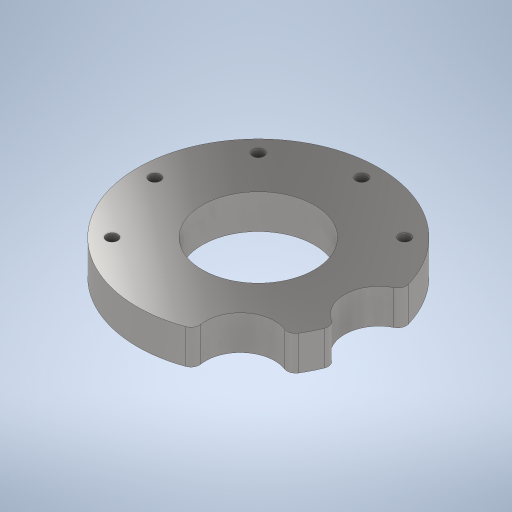
# Autodesk Inventor part: Weapon Hub Support
Saved by Autodesk Inventor 2023 (Build 270158000, 158)
## iProperties
Created: 2021-11-28
Part Number: Weapon Hub Support
Material: Steel, Carbon
Document SubType Name: Modeling
Designer: karen
Density: 7.85 g/cm^3
Appearance: Semi-Polished
Author: karen
Autodesk Inventor part; units mm, degrees
ref_plane "YZ Plane" through (0, 0, 0) normal (1, 0, 0) x (0, 1, 0)
ref_plane "XZ Plane" through (0, 0, 0) normal (0, 1, 0) x (-1, 0, 0)
ref_plane "XY Plane" through (0, 0, 0) normal (0, 0, 1) x (1, 0, 0)
sketch "Sketch1" plane through (0, 0, 0) normal (0, 1, 0) x (-1, 0, 0)
  circle A0 centre (0, 0) radius 44.45
  dimension "d0" = 88.9
  constraints: 1 centre point, 1 coincident
  measures "d0" diameter of A0
extrude "Extrusion1" add sketch "Sketch1" along normal blind 12.7
sketch "Sketch2" plane through (0, 12.7, 0) normal (0, 1, 0) x (1, 0, 0)
  circle A0 centre (0, 0) radius 19.05
  dimension "d3" = 38.1
  constraints: 1 centre point, 1 coincident
  measures "d3" diameter of A0
extrude "Extrusion2" cut sketch "Sketch2" against normal blind 12.7
sketch "Sketch4" plane through (0, 12.7, 0) normal (0, 1, 0) x (1, 0, 0)
  circle A0 centre (0, 0) radius 20.6375
  dimension "d17" = 41.275
  constraints: 1 centre point, 1 coincident
  measures "d17" diameter of A0
extrude "Extrusion4" cut sketch "Sketch4" against normal blind 25.4
sketch "Sketch5" plane through (0, 12.7, 0) normal (0, 1, 0) x (1, 0, 0)
  line L0 (0, 0) -> (0, 38.1)
  line L1 (0, 0) -> (26.9408, 26.9408)
  line L2 (0, 0) -> (-26.9408, 26.9408)
  line L3 (0, 0) -> (-38.1, 0)
  line L4 (0, 0) -> (-26.9408, -26.9408)
  circle A0 centre (0, 38.1) radius 2.0828
  circle A1 centre (26.9408, 26.9408) radius 2.0828
  circle A2 centre (-26.9408, 26.9408) radius 2.0828
  circle A3 centre (-38.1, 0) radius 2.0828
  circle A4 centre (-26.9408, -26.9408) radius 2.0828
  dimension "d20" = 38.1
  dimension "d21" = 38.1
  dimension "d22" = 45
  dimension "d23" = 38.1
  dimension "d24" = 45
  dimension "d25" = 38.1
  dimension "d26" = 38.1
  dimension "d27" = 45
  dimension "d28" = 4.1656
  dimension "d29" = 4.1656
  dimension "d30" = 4.1656
  dimension "d31" = 4.1656
  dimension "d32" = 4.1656
  constraints: 10 end point, 5 centre point, 4 coincident, 1 horizontal, 1 point on line, 1 vertical
  measures "d20" distance of L0.start L0.end
  measures "d21" distance of L0.start L1.end
  measures "d22" angle of L0 L1
  measures "d23" distance of L0.start L2.end
  measures "d24" angle of L0 L2
  measures "d25" distance of L0.start L3.end
  measures "d26" distance of L0.start L4.end
  measures "d27" angle of L3 L4
  measures "d28" diameter of A0
  measures "d29" diameter of A1
  measures "d30" diameter of A2
  measures "d31" diameter of A3
  measures "d32" diameter of A4
extrude "Extrusion5" cut sketch "Sketch5" against normal blind 12.7
sketch "Sketch6" plane through (0, 12.7, 0) normal (0, 1, 0) x (1, 0, 0)
  circle A0 centre (46.8049, -2.3327) radius 4.7625
  circle A1 centre (26.9408, 26.9408) radius 2.0828 projected
  point P0 (0, 0)
  dimension "d35" = 9.525
  dimension "d36" = 46.863
  dimension "d39" = 29.2735
  constraints: 1 centre point
  measures "d35" diameter of A0
  measures "d36" distance of point (0, 0) A0.centre
  measures "d39" vertical distance of A1.centre A0.centre
extrude "Extrusion6" cut sketch "Sketch6" against normal blind 12.7 contours A0
sketch "Sketch7" plane through (0, 12.7, 0) normal (0, 1, 0) x (1, 0, 0)
  circle A0 centre (29.6672, -36.322) radius 4.7625
  point P0 (0, 0)
  dimension "d40" = 9.525
  dimension "d41" = 29.6672
  dimension "d42" = 36.322
  constraints: 1 centre point
  measures "d40" diameter of A0
  measures "d41" horizontal distance of point (0, 0) A0.centre
  measures "d42" vertical distance of point (0, 0) A0.centre
extrude "Extrusion7" cut sketch "Sketch7" against normal blind 12.7
sketch "Sketch8" plane through (0, 12.7, 0) normal (0, 1, 0) x (1, 0, 0)
  arc A0 (31.0831, -31.7749) -> (24.9289, -36.8015) centre (29.6672, -36.322) ccw projected
  circle A1 centre (29.6672, -36.322) radius 12.7
  arc A2 (44.4141, 1.7862) -> (44.0164, -6.1935) centre (46.8049, -2.3327) ccw projected
  circle A3 centre (46.8049, -2.3327) radius 12.7
  point P0 (0, 0)
  dimension "d45" = 25.4
  dimension "d46" = 25.4
  constraints: 2 centre point, 2 coincident
  measures "d45" diameter of A1
  measures "d46" diameter of A3
extrude "Extrusion8" cut sketch "Sketch8" against normal blind 12.7
fillet "Fillet1" radius 3.175 4 edges at (43.337, 6.35, -9.8846) (42.1394, 6.35, 14.1447) (36.3795, 6.35, 25.5408) (17.7629, 6.35, 40.7466)
body "Solid1"
